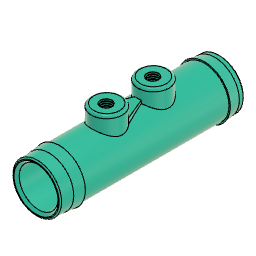
venturi-3-4 (Autodesk Fusion 360 design; units mm, degrees)
Autodesk Fusion 360 part; units mm, degrees
sketch "Sketch1" plane through (0, 0, 0) normal (0, 1, 0) x (1, 0, 0)
  circle A0 centre (0, 0) radius 11
  dimension "d1" = 22
  constraint coincident A0.centre origin
  measures "d1" diameter of A0
sketch "Sketch2" plane through (0, 0, 0) normal (1, 0, 0) x (0, 1, 0)
  line L0 (0, 0) -> (71, 0) construction
  line L1 (70.5166, 9.4747) -> (69, 9.525)
  line L2 (5, 9.525) -> (0.4834, 9.3752)
  line L3 (0, 8.8754) -> (0, 7.525)
  line L4 (0, 7.525) -> (29.6309, 7.525)
  line L5 (29.6309, 7.525) -> (42.0066, 3.0206)
  line L6 (42.6907, 2.9) -> (47.919, 2.9)
  line L7 (48.3519, 2.9474) -> (69, 7.525)
  line L8 (69, 7.525) -> (71, 7.525)
  line L9 (71, 8.975) -> (71, 7.525)
  line L10 (0, 7.525) -> (0, 0) construction
  line L11 (9, 9.525) -> (65, 9.525)
  line L12 (71, 0) -> (71, 7.525) construction
  arc A0 (42.0066, 3.0206) -> (42.6907, 2.9) centre (42.6907, 4.9) ccw
  arc A1 (47.919, 2.9) -> (48.3519, 2.9474) centre (47.919, 4.9) ccw
  arc A2 (0.4834, 9.3752) -> (0, 8.8754) centre (0.5, 8.8754) ccw
  arc A3 (71, 8.975) -> (70.5166, 9.4747) centre (70.5, 8.975) ccw
  line L13 (69, 7.525) -> (69, 0) construction
  line L14 (29.6309, 7.525) -> (29.6309, 0) construction
  line L15 (69, 9.525) -> (65, 10.025)
  line L16 (65, 10.025) -> (65, 9.525)
  line L17 (65, 9.525) -> (69, 9.525) construction
  line L18 (5, 9.525) -> (9, 10.025)
  line L19 (9, 10.025) -> (9, 9.525)
  line L20 (9, 9.525) -> (5, 9.525) construction
  point P0 (71, 9.4587)
  point P1 (0, 9.3591)
  point P2 (42.338, 2.9)
  point P3 (48.138, 2.9)
  dimension "d60" = 20
  dimension "d61" = 2.9
  dimension "d62" = 5.8
  dimension "d63" = 12.5
  dimension "d66" = 2
  dimension "d67" = 2
  dimension "d68" = 0.5
  dimension "d69" = 0.5
  dimension "d72" = 2
  dimension "d74" = 2
  dimension "d75" = 1.9
  dimension "d77" = 5
  dimension "d78" = 1.9
  dimension "d81" = 9.525
  dimension "d84" = 2
  dimension "d85" = 5.9375
  dimension "d94" = 4
  dimension "d95" = 0.5
  dimension "d96" = 0.5
  dimension "d97" = 4
  dimension "d107" = 71
  constraint coincident L0.start L10.end
  constraint horizontal L0
  constraint perpendicular L3 L4
  constraint perpendicular L3 L6
  constraint perpendicular L0 L10
  constraint vertical L9
  constraint horizontal L8
  constraint vertical L1.end L7.end
  constraint vertical L12
  constraint coincident P2 L5
  constraint coincident P2 L6
  constraint tangent L5 A0
  constraint tangent L6 A0
  constraint coincident P3 L6
  constraint coincident P3 L7
  constraint tangent L6 A1
  constraint tangent L7 A1
  constraint coincident P1 L2
  constraint coincident P1 L3
  constraint tangent L2 A2
  constraint tangent L3 A2
  constraint coincident P0 L1
  constraint coincident P0 L9
  constraint tangent L1 A3
  constraint tangent L9 A3
  constraint horizontal L11
  constraint coincident L0 L13.end
  constraint perpendicular L0 L13
  constraint coincident L0 L14.end
  constraint perpendicular L0 L14
  constraint perpendicular L11 L16
  constraint horizontal L17
  constraint perpendicular L11 L19
  constraint perpendicular L19 L20
  measures "d60" angle of L0 L5
  measures "d61" distance of L0 L6
  measures "d62" distance of P2 P3
  measures "d63" angle of L6 L7
  measures "d66" radius of A0
  measures "d67" radius of A1
  measures "d68" radius of A2
  measures "d69" radius of A3
  measures "d72" distance of L7.end L8.end
  measures "d74" distance of L1.end L7.end
  measures "d75" angle of L1 L8
  measures "d77" horizontal distance of L2.start L3.end
  measures "d78" angle of L2 L4
  measures "d81" distance of L0 L11
  measures "d84" distance of L4 L11
  measures "d94" distance of L1.end L16
  measures "d95" distance of L15.end L11.end
  measures "d96" distance of L18.end L11.start
  measures "d97" distance of L2.start L19
  measures "d107" distance of L3 L9
sketch "Sketch14" plane through (0, 0, 0) normal (0, 0, 1) x (1, 0, 0)
  line L0 (0, 45.3048, 2.9) -> (9, 45.3048, 2.9)
  line L1 (0, 42.6907, 2.9) -> (0, 47.919, 2.9)
revolve "Revolve1" add sketch "Sketch2" angle 360 about axis through (0, 0, 0) along (0, 1, 0)
ref_plane "WorkPlane1" through (0, 48.26, 0) normal (0, -1, 0) x (0, 0, -1)
sketch "Sketch4" plane through (0, 0, 0) normal (0, 0, 1) x (1, 0, 0)
  circle A0 centre (0, 45.3048) radius 1
  circle A1 centre (0, 27.3048) radius 1
  line L0 (0, 45.3048) -> (9, 45.3048)
  dimension "d22" = 2
  dimension "d108" = 18
  constraint equal A0 A1
  constraint vertical origin A0.centre
  constraint vertical origin A1.centre
  constraint coincident A0.centre L0
  measures "d22" diameter of A0
  measures "d108" distance of A0.centre A1.centre
extrude "Extrude1" cut sketch "Sketch4" along normal blind 12.7
ref_plane "WorkPlane2" through (0, 0, 4.445) normal (0, 0, 1) x (1, 0, 0)
sketch "Sketch5" plane through (0, 0, 4.445) normal (0, 0, 1) x (1, 0, 0)
ref_plane "WorkPlane3" through (0, 0, 15) normal (0, 0, 1) x (1, 0, 0)
sketch "Sketch9" plane through (0, 0, 15) normal (0, 0, 1) x (1, 0, 0)
  circle A0 centre (0, 45.3048) radius 6
  circle A1 centre (0, 27.3048) radius 6
  circle A2 centre (0, 27.3048) radius 1.5
  circle A3 centre (0, 45.3048) radius 1.5
  point P0 (0, 27.3048)
  point P1 (0, 45.3048)
  dimension "d47" = 12
  dimension "d49" = 3
  dimension "d83" = 3
  constraint equal A0 A1
  constraint concentric A1 A2
  constraint concentric A0 A3
  constraint coincident P0 A1.centre
  constraint coincident A0.centre A3.centre
  measures "d47" diameter of A0
  measures "d49" diameter of A3
  measures "d83" diameter of A2
extrude "Extrude7" add sketch "Sketch9" along normal up to surface contours A0 end surface at (-2.2129, 39.7486, 9.2644)
sketch "Sketch10" plane through (0, 0, 0) normal (0, 0, 1) x (1, 0, 0)
sketch "Sketch11" plane through (0, 0, 0) normal (1, 0, 0) x (0, 1, 0)
sketch "Sketch12" plane through (0, 0, 0) normal (0, 1, 0) x (1, 0, 0)
sketch "Sketch13" plane through (0, 0, 0) normal (0, -1, 0) x (1, 0, 0)
  circle A0 centre (0, 0) radius 7.525
  circle A1 centre (0, 0) radius 8.8754
extrude "Extrude9" add sketch "Sketch9" along normal up to surface contours A1 end surface at (-7.0001, 39.7516, 6.4595)
ref_plane "WorkPlane4" through (0, 10.5147, 9.525) normal (0, 0, 1) x (-1, 0, 0)
sketch "Sketch15" plane through (0, 14.8767, 9.525) normal (0, 0, 1) x (-1, 0, 0)
  line L0 (0, -27.4281) -> (5, -15.4281)
  line L1 (5, -15.4281) -> (-5, -15.4281)
  line L2 (-5, -15.4281) -> (0, -27.4281)
  line L3 (0, -27.4281) -> (0, -15.4281)
  line L4 (0, 5.8767) -> (0, -50.1233)
  circle A0 centre (0, -30.4281) radius 6
  circle A1 centre (0, -12.4281) radius 6
  point P0 (0, -12.4281)
  point P1 (0, -30.4281)
  dimension "d109" = 3
  dimension "d110" = 10
  dimension "d111" = 3
  constraint horizontal L1
  constraint coincident L1 L3.end
  constraint midpoint L1 L3.end
  constraint coincident L0.start L4
  constraint coincident L3.end L4
  measures "d109" distance of L3.end P0
  measures "d110" distance of L0.end L1.end
  measures "d111" distance of L0.start A0.centre
extrude "Extrude10" add sketch "Sketch15" along normal blind 1 and the other way blind 1 contours L0 L3 L4 A0 | L2 L3 L4 A0 | L0 L3 L4 A0 A1 | L2 L3 L4 A0 A1 | L0 L1 L3 L4 A1 | L1 L2 L3 L4 A1
hole "Hole1" at (0, 45.3048, 15) direction (0, 0, -1) diameter 4.064 depth 7 tip angle 180
thread "Thread1" "ANSI Unified Screw Threads 0.19(#10) 10-32 UNF 2B" major diameter 4.826 minor diameter 4.064 pitch 0.7937 angle 60 modelled right hand crest width 0.2253 on face at (0.2023, 43.2829, 12.6667) crest through (2.032, 45.3048, 14.8016)
hole "Hole2" at (0, 27.3048, 15) direction (0, 0, -1) diameter 3.823 depth 5.5 tip angle 180
thread "Thread2" "ANSI Unified Screw Threads 0.19(#10) 10-32 UNF 2B" major diameter 4.826 minor diameter 4.064 pitch 0.7937 angle 60 modelled right hand crest width 0.2253 on face at (0.0953, 25.3957, 13.1667) crest through (2.032, 27.3048, 14.8016)
fillet "Fillet1" radius 1 2 edges at (-5.594, 43.1351, 15) (-5.594, 25.1351, 15)
chamfer "Chamfer1" distance 1 angle 45 1 edges at (-7.0158, 0, 2.7212)
equation "d61 = ( 5.8 / 2 ) * 1 mm"
equation "d62 = d61 * 2"
equation "d81 = ( 19.05 / 2 ) * 1 mm"
equation "d83 = d49"
